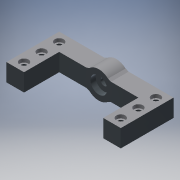
# Autodesk Inventor part: Block1
Saved by Autodesk Inventor 2016 (Build 200138000, 138)
## iProperties
Created: 2015-06-05
Part Number: Block1
Material: Générique
Document SubType Name: Modeling
Designer: Logan
Density: 1 g/cm^3
Appearance: Par défaut
Author: Logan
Autodesk Inventor part; units mm, degrees
ref_plane "YZ Plane" through (0, 0, 0) normal (1, 0, 0) x (0, 1, 0)
ref_plane "XZ Plane" through (0, 0, 0) normal (0, 1, 0) x (-1, 0, 0)
ref_plane "XY Plane" through (0, 0, 0) normal (0, 0, 1) x (1, 0, 0)
sketch "Esquisse8" plane through (0, 0, 0) normal (0, 0, 1) x (1, 0, 0)
  line L0 (65, -20) -> (65, 40)
  line L1 (65, 40) -> (-65, 40)
  line L2 (-65, 40) -> (-65, -20)
  line L3 (-45, 20) -> (45, 20)
  line L4 (-45, 20) -> (-45, -20)
  line L5 (45, 20) -> (45, -20)
  line L6 (65, -20) -> (45, -20)
  line L7 (-45, -20) -> (-65, -20)
  point P0 (0, 0)
  dimension "d45" = 20
  dimension "d46" = 90
  dimension "d47" = 45
  dimension "d71" = 20
  dimension "d72" = 20
  constraints: 16 end point, 2 perpendicular, 1 collinear, 1 parallel
  measures "d45" distance between parallel lines of L1 L3
  measures "d46" distance between parallel lines of L5 L4
  measures "d47" distance from line of point (0, 0) L4
  measures "d71" distance from line of point (0, 0) L3
  measures "d72" distance from line of point (0, 0) L6
extrude "Extrusion7" add sketch "Esquisse8" along normal blind 60
sketch "Esquisse10" plane through (0, 0, 0) normal (0, 0, -1) x (-1, 0, 0)
  line L0 (45, 20) -> (-45, 20) projected
  line L1 (-55, 30) -> (-55, 10)
  line L2 (55, 10) -> (55, 30)
  line L3 (-55, 10) -> (-55, -10)
  line L4 (55, 10) -> (55, -10)
  dimension "d75" = 20
  dimension "d80" = 20
  dimension "d89" = 20
  dimension "d90" = 20
  constraints: 8 end point, 2 vertical
  measures "d75" distance of L1.start L1.end
  measures "d80" distance of L2.start L2.end
  measures "d89" distance of L1.end L3.end
  measures "d90" distance of L2.start L4.end
hole "Perçage2" at (55, 10, 0) at (-55, 10, 0) at (-55, 30, 0) at (55, 30, 0) at (-55, -10, 0) at (55, -10, 0) direction (0, 0, 1) diameter 6 end through all counterbore diameter 10 counterbore depth 4
sketch "Esquisse13" plane through (-65, 40, 0) normal (0, 1, 0) x (1, 0, 0)
  line L0 (65, 0) -> (65, -20)
  circle A0 centre (65, -20) radius 4
  dimension "d81" = 20
  dimension "d82" = 8
  constraints: 2 end point, 1 centre point, 1 coincident, 1 vertical
  measures "d81" distance of L0.start L0.end
  measures "d82" diameter of A0
extrude "Extrusion9" cut sketch "Esquisse13" against normal up to surface (20 mm away)
sketch "Esquisse14" plane through (-65, 40, 0) normal (0, 1, 0) x (1, 0, 0)
  circle A0 centre (65, -20) radius 4 projected
  line L0 (0, 0) -> (130, 0) projected
  line L1 (0, 0) -> (0, -60) projected
  line L2 (130, -60) -> (0, -60) projected
  line L3 (130, 0) -> (130, -60) projected
  circle A1 centre (65, -20) radius 9.5
  point P0 (65, 0)
  dimension "d85" = 19
  constraints: 1 centre point, 1 coincident
  measures "d85" diameter of A1
extrude "Extrusion10" cut sketch "Esquisse14" against normal blind 6 contours A1
ref_plane "Plan de construction3" through (-65, 30, 0) normal (0, 1, 0) x (1, 0, 0)
mirror "Symétrie5" about plane through (-65, 30, 0) normal (0, 1, 0) of "Extrusion10"
sketch "Esquisse15" plane through (-65, 40, 0) normal (0, 1, 0) x (1, 0, 0)
  circle A0 centre (65, -20) radius 9.5 projected
  circle A1 centre (65, -20) radius 15.5
  line L0 (130, -60) -> (0, -60) projected
  line L1 (0, 0) -> (130, 0) projected
  line L2 (130, 0) -> (130, -10)
  line L3 (130, -30) -> (130, -60)
  line L4 (0, 0) -> (0, -10)
  line L5 (0, -30) -> (0, -60)
  line L6 (130, -30) -> (76.8427, -30)
  line L7 (53.1573, -30) -> (0, -30)
  line L8 (0, -10) -> (53.1573, -10)
  line L9 (76.8427, -10) -> (130, -10)
  point P0 (65, 0)
  dimension "d91" = 6
  constraints: 16 end point, 4 parallel, 4 point on circle, 1 centre point
  measures "d91" radial gap between concentric circles of A0 A1
extrude "Extrusion11" cut sketch "Esquisse15" against normal through all contours A1 L8 L4 L1 L2 L9 | L6 L3 L0 L5 L7 A1
sketch "Esquisse16" plane through (65, 40, 10) normal (0, 0, -1) x (-1, 0, 0)
  circle A0 centre (10, -50) radius 3 projected
  circle A1 centre (10, -30) radius 3 projected
  circle A2 centre (10, -10) radius 3 projected
  circle A3 centre (120, -10) radius 3 projected
  circle A4 centre (120, -30) radius 3 projected
  circle A5 centre (120, -50) radius 3 projected
  circle A6 centre (10, -50) radius 5
  circle A7 centre (10, -30) radius 5
  circle A8 centre (10, -10) radius 5
  circle A9 centre (120, -10) radius 5
  circle A10 centre (120, -30) radius 5
  circle A11 centre (120, -50) radius 5
  point P0 (65, -40)
  dimension "d96" = 10
  dimension "d97" = 10
  constraints: 6 centre point, 4 equal radius
  measures "d96" diameter of A6
  measures "d97" diameter of A7
extrude "Extrusion12" cut sketch "Esquisse16" against normal blind 4 contours A0 | A1 | A2 | A3 | A4 | A5 | A6 | A7 | A8 | A9 | A10 | A11
ref_plane "Plan de construction4" through (11.8427, 40, 20) normal (0, 0, 1) x (1, 0, 0)
mirror "Symétrie6" about plane through (11.8427, 40, 20) normal (0, 0, 1) of "Extrusion12"
chamfer "Chanfrein1" distance 2 angle 45 4 edges at (11.8427, 30, 10) (11.8427, 30, 30) (-11.8427, 30, 30) (-11.8427, 30, 10)
